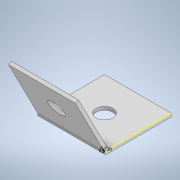
# Autodesk Inventor part: trail 17
Saved by Autodesk Inventor 2020.2 (Build 242310000, 310)
## iProperties
Created: 2020-03-01
Part Number: trail 17
Material: Generic
Document SubType Name: Modeling
Designer: lenovo
Density: 1 g/cm^3
Appearance: Default
Author: lenovo
Autodesk Inventor part; units mm, degrees
ref_plane "YZ Plane" through (0, 0, 0) normal (1, 0, 0) x (0, 1, 0)
ref_plane "XZ Plane" through (0, 0, 0) normal (0, 1, 0) x (-1, 0, 0)
sketch "Sketch1" plane through (0, 0, 0) normal (0, 1, 0) x (-1, 0, 0)
  line L0 (-10, -10) -> (10, -10)
  line L1 (10, -10) -> (10, 10)
  line L2 (10, 10) -> (-10, 10)
  line L3 (-10, 10) -> (-10, -10)
  line L4 (-10, -10) -> (10, 10) construction
  line L5 (10, -10) -> (-10, 10) construction
  point P0 (0, 0)
  dimension "d0" = 20
  dimension "d1" = 20
  constraints: 12 end point, 2 midpoint, 2 parallel, 1 horizontal, 1 perpendicular
  measures "d0" distance of L2.end L1.end
  measures "d1" distance of L1.end L0.end
extrude "Extrusion1" add sketch "Sketch1" along normal blind 1
sketch "Sketch3" plane through (10, 0, 10) normal (1, 0, 0) x (0, 0, -1)
  line L0 (20, 1) -> (0, 1) projected
  line L1 (0, 1) -> (-0.9142, 2.7788)
  line L2 (0, 1) -> (2, 1) construction
  point P0 (10, 0)
  dimension "d5" = 2
  dimension "d6" = 117.2
  constraints: 4 end point, 1 equal length, 1 horizontal
  measures "d5" distance of L0.end L1.end
  measures "d6" angle of L2 L1
ref_plane "Work Plane1" through (10, 1, 10) normal (0, 0.4570979, -0.8894164) x (0, 0.8894164, 0.4570979)
sketch "Sketch4" plane through (10, 1, 10) normal (0, 0.4570979, -0.8894164) x (0, 0.8894164, 0.4570979)
  line L0 (-9.142, -20) -> (0, -20) projected
  line L1 (0, -20) -> (19, -20)
  line L2 (19, -20) -> (19, 0)
  line L3 (19, 0) -> (0, 0)
  line L4 (0, 0) -> (0, -20)
  point P0 (-5.4604, -10)
  dimension "d7" = 19
  dimension "d8" = 20
  constraints: 8 end point, 2 parallel, 1 horizontal, 1 perpendicular
  measures "d7" distance of L3.end L2.end
  measures "d8" distance of L2.end L1.end
extrude "Extrusion2" add sketch "Sketch4" along normal blind 1
sketch "Sketch5" plane through (10, 1, 10) normal (1, 0, 0) x (0, 0.4570979, -0.8894164)
  line L0 (0, 0) -> (1, 0) projected
  line L1 (1, 0) -> (1, -0.5139)
  line L2 (17.7883, -9.142) -> (0, 0) projected
  line L3 (1, 0) -> (0, 0)
  line L4 (0, 0) -> (1, -0.5139)
  point P0 (8.4371, -5.4604)
  constraints: 6 end point, 2 point on line, 1 collinear, 1 vertical
extrude "Extrusion3" add sketch "Sketch5" against normal blind 20
fillet "Fillet1" radius 0.5 2 edges at (0, 1, 8.8757) (0, 0, 10)
sketch "Sketch6" plane through (0, 1, 0) normal (0, 1, 0) x (1, 0, 0)
  circle A0 centre (0, 0) radius 2.5
  dimension "d14" = 5
  constraints: 1 centre point, 1 coincident
  measures "d14" diameter of A0
sketch "Sketch7" plane through (10, 1.4571, 9.1106) normal (0, 0.4570979, -0.8894164) x (-1, 0, 0)
  circle A0 centre (10, 9.5) radius 2.5
  point P0 (10, -5.4604)
  dimension "d15" = 5
  constraints: 1 centre point
  measures "d15" diameter of A0
extrude "Extrusion4" cut sketch "Sketch6" against normal blind 10
extrude "Extrusion5" cut sketch "Sketch7" against normal blind 10
body "Solid1"
